Autodesk Fusion 360 part; units mm, degrees
(part 2 of 2)
  arc A403 (168.143, 73.5075) -> (169.394, 73.446) centre (168.77, 73.5075) ccw
  line L397 (168.143, 73.5075) -> (168.146, 74.619)
  circle A404 centre (161.56, 73.5325) radius 0.325
  circle A405 centre (167.34, 73.5325) radius 0.325
  arc A406 (174.75, 72.525) -> (175, 72.775) centre (174.75, 72.775) ccw
  line L398 (174.75, 72.525) -> (173.85, 72.525)
  arc A407 (173.6, 72.775) -> (173.85, 72.525) centre (173.85, 72.775) ccw
  line L399 (173.6, 72.775) -> (173.6, 73.3)
  arc A408 (173.85, 73.55) -> (173.6, 73.3) centre (173.85, 73.3) ccw
  line L400 (173.85, 73.55) -> (174.75, 73.55)
  arc A409 (175, 73.3) -> (174.75, 73.55) centre (174.75, 73.3) ccw
  line L401 (175, 73.3) -> (175, 72.775)
  arc A410 (157.05, 72.475) -> (157.3, 72.725) centre (157.05, 72.725) ccw
  line L402 (157.05, 72.475) -> (156.15, 72.475)
  arc A411 (155.9, 72.725) -> (156.15, 72.475) centre (156.15, 72.725) ccw
  line L403 (155.9, 72.725) -> (155.9, 73.25)
  arc A412 (156.15, 73.5) -> (155.9, 73.25) centre (156.15, 73.25) ccw
  line L404 (156.15, 73.5) -> (157.05, 73.5)
  arc A413 (157.3, 73.25) -> (157.05, 73.5) centre (157.05, 73.25) ccw
  line L405 (157.3, 73.25) -> (157.3, 72.725)
  arc A414 (174.775, 70) -> (175.025, 70.25) centre (174.775, 70.25) ccw
  line L406 (174.775, 70) -> (173.825, 70)
  arc A415 (173.575, 70.25) -> (173.825, 70) centre (173.825, 70.25) ccw
  line L407 (173.575, 70.25) -> (173.575, 70.75)
  arc A416 (173.825, 71) -> (173.575, 70.75) centre (173.825, 70.75) ccw
  line L408 (173.825, 71) -> (174.775, 71)
  arc A417 (175.025, 70.75) -> (174.775, 71) centre (174.775, 70.75) ccw
  line L409 (175.025, 70.75) -> (175.025, 70.25)
  arc A418 (160.632, 70.2525) -> (159.628, 70.2525) centre (160.13, 70.2525) ccw
  line L410 (160.632, 70.2525) -> (160.632, 69.4525)
  arc A419 (159.628, 69.4525) -> (160.632, 69.4525) centre (160.13, 69.4525) ccw
  line L411 (159.628, 69.4525) -> (159.628, 70.2525)
  arc A420 (169.272, 70.2525) -> (168.268, 70.2525) centre (168.77, 70.2525) ccw
  line L412 (169.272, 70.2525) -> (169.272, 69.4525)
  arc A421 (168.268, 69.4525) -> (169.272, 69.4525) centre (168.77, 69.4525) ccw
  line L413 (168.268, 69.4525) -> (168.268, 70.2525)
  arc A422 (174.775, 68.1) -> (175.025, 68.35) centre (174.775, 68.35) ccw
  line L414 (174.775, 68.1) -> (173.825, 68.1)
  arc A423 (173.575, 68.35) -> (173.825, 68.1) centre (173.825, 68.35) ccw
  line L415 (173.575, 68.35) -> (173.575, 68.85)
  arc A424 (173.825, 69.1) -> (173.575, 68.85) centre (173.825, 68.85) ccw
  line L416 (173.825, 69.1) -> (174.775, 69.1)
  arc A425 (175.025, 68.85) -> (174.775, 69.1) centre (174.775, 68.85) ccw
  line L417 (175.025, 68.85) -> (175.025, 68.35)
  line L418 (220, 60) -> (110, 60)
  line L419 (110, 60) -> (110, 170)
  line L420 (110, 170) -> (220, 170)
  line L421 (220, 170) -> (220, 60)
  line L422 (220, 60) -> (110, 170) construction
  line L423 (110, 60) -> (220, 170) construction
  point P0 (165, 115)
  constraint horizontal L418
  constraint perpendicular L418 L419
  constraint parallel L418 L420
  constraint parallel L419 L421
  constraint coincident L422 P0
  constraint coincident L423 P0
extrude "Extrude1" add sketch "Sketch1" along normal blind 10 contours L418 L419 L420 L421
sketch "Sketch2" plane through (0, 0, -0.05) normal (0, 0, 1) x (-1, 0, 0)
  line L0 (-115.9, 71.8) -> (-115.9024, 71.5818)
  arc A0 (-120.6818, 66.8024) -> (-115.9024, 71.5818) centre (-120.9, 71.8) ccw
  line L1 (-120.6818, 66.8024) -> (-120.9, 66.8)
  line L2 (-120.9, 66.8) -> (-209.95, 66.8)
  line L3 (-209.95, 66.8) -> (-210.1682, 66.8024)
  arc A1 (-214.9476, 71.5818) -> (-210.1682, 66.8024) centre (-209.95, 71.8) ccw
  line L4 (-214.9476, 71.5818) -> (-214.95, 71.8)
  line L5 (-214.95, 71.8) -> (-214.95, 155.9)
  line L6 (-214.95, 155.9) -> (-214.9476, 156.1182)
  arc A2 (-210.1682, 160.8976) -> (-214.9476, 156.1182) centre (-209.95, 155.9) ccw
  line L7 (-210.1682, 160.8976) -> (-209.95, 160.9)
  line L8 (-209.95, 160.9) -> (-120.9, 160.9)
  line L9 (-120.9, 160.9) -> (-120.6818, 160.8976)
  arc A3 (-115.9024, 156.1182) -> (-120.6818, 160.8976) centre (-120.9, 155.9) ccw
  line L10 (-115.9024, 156.1182) -> (-115.9, 155.9)
  line L11 (-115.9, 155.9) -> (-115.9, 71.8)
  line L12 (-110, 170) -> (-220, 170)
  line L13 (-220, 170) -> (-220, 60)
  line L14 (-220, 60) -> (-110, 60)
  line L15 (-110, 60) -> (-110, 170)
  circle A4 centre (-122.6756, 73.6401) radius 7.5719
  circle A5 centre (-208.2, 73.5) radius 7.6609
  circle A6 centre (-211.7862, 157.3826) radius 8.1229
  circle A7 centre (-122.6, 154.1) radius 8.9766
extrude "Extrude2" add sketch "Sketch2" against normal blind 10 contours L0 A0 L1 L2 L11 A4 | L8 L9 A3 L10 L11 A7 | L2 L3 A1 L4 L5 A5 | L5 L6 A2 L7 L8 A6 picked at (-121.8657, 72.2322) picked at (-121.9336, 154.8688) picked at (-209.4122, 72.673) picked at (-210.1646, 156.3085)
sketch "Sketch3" plane through (0, 0, -10.05) normal (0, 0, -1) x (1, 0, 0)
  line L0 (115.9, 77.02) -> (115.9, 148.126)
  arc A0 (115.9, 148.126) -> (128.4599, 160.9) centre (122.6, 154.1) ccw
  line L1 (128.4599, 160.9) -> (204.4644, 160.9)
  arc A1 (204.4644, 160.9) -> (214.95, 149.9011) centre (211.7862, 157.3826) ccw
  line L2 (214.95, 149.9011) -> (214.95, 77.1232)
  arc A2 (214.95, 77.1232) -> (204.4852, 66.8) centre (208.2, 73.5) ccw
  line L3 (204.4852, 66.8) -> (125.9231, 66.8)
  arc A3 (125.9231, 66.8) -> (115.9, 77.02) centre (122.6756, 73.6401) ccw
  line L4 (220, 170) -> (110, 170)
  line L5 (110, 170) -> (110, 60)
  line L6 (110, 60) -> (220, 60)
  line L7 (220, 60) -> (220, 170)
sketch "Sketch4" plane through (0, 0, 1.56) normal (0, 0, 1) x (-1, 0, 0)
  arc A0 (-120.6818, 66.8024) -> (-115.9024, 71.5818) centre (-120.9, 71.8) ccw
  line L0 (-115.9024, 71.5818) -> (-115.9, 71.8)
  line L1 (-115.9, 71.8) -> (-115.9, 155.9)
  line L2 (-115.9, 155.9) -> (-115.9024, 156.1182)
  arc A1 (-115.9024, 156.1182) -> (-120.6818, 160.8976) centre (-120.9, 155.9) ccw
  line L3 (-120.6818, 160.8976) -> (-120.9, 160.9)
  line L4 (-120.9, 160.9) -> (-209.95, 160.9)
  line L5 (-209.95, 160.9) -> (-210.1682, 160.8976)
  arc A2 (-210.1682, 160.8976) -> (-214.9476, 156.1182) centre (-209.95, 155.9) ccw
  line L6 (-214.9476, 156.1182) -> (-214.95, 155.9)
  line L7 (-214.95, 155.9) -> (-214.95, 71.8)
  line L8 (-214.95, 71.8) -> (-214.9476, 71.5818)
  arc A3 (-214.9476, 71.5818) -> (-210.1682, 66.8024) centre (-209.95, 71.8) ccw
  line L9 (-210.1682, 66.8024) -> (-209.95, 66.8)
  line L10 (-209.95, 66.8) -> (-120.9, 66.8)
  line L11 (-120.9, 66.8) -> (-120.6818, 66.8024)
  circle A4 centre (-122.55, 154.05) radius 2.2
  circle A5 centre (-208.4, 153.95) radius 2.2
  circle A6 centre (-165.24, 143.58) radius 2
  circle A7 centre (-160.16, 143.58) radius 0.85
  circle A8 centre (-170.32, 143.58) radius 0.85
  circle A9 centre (-161.43, 141.04) radius 1.1
  circle A10 centre (-167.78, 138.5) radius 1.1
  arc A11 (-139.5592, 132.4456) -> (-139.2145, 132.4456) centre (-139.3868, 132.6179) ccw
  line L12 (-139.5592, 132.4456) -> (-140.2044, 133.0908)
  arc A12 (-140.2044, 133.4355) -> (-140.2044, 133.0908) centre (-140.0321, 133.2632) ccw
  line L13 (-140.2044, 133.4355) -> (-139.8597, 133.7802)
  arc A13 (-139.515, 133.7802) -> (-139.8597, 133.7802) centre (-139.6873, 133.6079) ccw
  line L14 (-139.515, 133.7802) -> (-138.8698, 133.135)
  arc A14 (-138.8698, 132.7903) -> (-138.8698, 133.135) centre (-139.0421, 132.9627) ccw
  line L15 (-138.8698, 132.7903) -> (-139.2145, 132.4456)
  arc A15 (-134.6092, 132.3956) -> (-134.2645, 132.3956) centre (-134.4368, 132.5679) ccw
  line L16 (-134.6092, 132.3956) -> (-135.2544, 133.0408)
  arc A16 (-135.2544, 133.3855) -> (-135.2544, 133.0408) centre (-135.0821, 133.2132) ccw
  line L17 (-135.2544, 133.3855) -> (-134.9097, 133.7302)
  arc A17 (-134.565, 133.7302) -> (-134.9097, 133.7302) centre (-134.7373, 133.5579) ccw
  line L18 (-134.565, 133.7302) -> (-133.9198, 133.085)
  arc A18 (-133.9198, 132.7403) -> (-133.9198, 133.085) centre (-134.0921, 132.9127) ccw
  line L19 (-133.9198, 132.7403) -> (-134.2645, 132.3956)
  arc A19 (-129.8592, 132.2456) -> (-129.5145, 132.2456) centre (-129.6868, 132.4179) ccw
  line L20 (-129.8592, 132.2456) -> (-130.5044, 132.8908)
  arc A20 (-130.5044, 133.2355) -> (-130.5044, 132.8908) centre (-130.3321, 133.0632) ccw
  line L21 (-130.5044, 133.2355) -> (-130.1597, 133.5802)
  arc A21 (-129.815, 133.5802) -> (-130.1597, 133.5802) centre (-129.9873, 133.4079) ccw
  line L22 (-129.815, 133.5802) -> (-129.1698, 132.935)
  arc A22 (-129.1698, 132.5903) -> (-129.1698, 132.935) centre (-129.3421, 132.7627) ccw
  line L23 (-129.1698, 132.5903) -> (-129.5145, 132.2456)
  arc A23 (-140.885, 131.1198) -> (-140.5403, 131.1198) centre (-140.7127, 131.2921) ccw
  line L24 (-140.885, 131.1198) -> (-141.5302, 131.765)
  arc A24 (-141.5302, 132.1097) -> (-141.5302, 131.765) centre (-141.3579, 131.9373) ccw
  line L25 (-141.5302, 132.1097) -> (-141.1855, 132.4544)
  arc A25 (-140.8408, 132.4544) -> (-141.1855, 132.4544) centre (-141.0132, 132.2821) ccw
  line L26 (-140.8408, 132.4544) -> (-140.1956, 131.8092)
  arc A26 (-140.1956, 131.4645) -> (-140.1956, 131.8092) centre (-140.3679, 131.6368) ccw
  line L27 (-140.1956, 131.4645) -> (-140.5403, 131.1198)
  arc A27 (-135.935, 131.0698) -> (-135.5903, 131.0698) centre (-135.7627, 131.2421) ccw
  line L28 (-135.935, 131.0698) -> (-136.5802, 131.715)
  arc A28 (-136.5802, 132.0597) -> (-136.5802, 131.715) centre (-136.4079, 131.8873) ccw
  line L29 (-136.5802, 132.0597) -> (-136.2355, 132.4044)
  arc A29 (-135.8908, 132.4044) -> (-136.2355, 132.4044) centre (-136.0632, 132.2321) ccw
  line L30 (-135.8908, 132.4044) -> (-135.2456, 131.7592)
  arc A30 (-135.2456, 131.4145) -> (-135.2456, 131.7592) centre (-135.4179, 131.5868) ccw
  line L31 (-135.2456, 131.4145) -> (-135.5903, 131.0698)
  arc A31 (-131.185, 130.9198) -> (-130.8403, 130.9198) centre (-131.0127, 131.0921) ccw
  line L32 (-131.185, 130.9198) -> (-131.8302, 131.565)
  arc A32 (-131.8302, 131.9097) -> (-131.8302, 131.565) centre (-131.6579, 131.7373) ccw
  line L33 (-131.8302, 131.9097) -> (-131.4855, 132.2544)
  arc A33 (-131.1408, 132.2544) -> (-131.4855, 132.2544) centre (-131.3132, 132.0821) ccw
  line L34 (-131.1408, 132.2544) -> (-130.4956, 131.6092)
  arc A34 (-130.4956, 131.2645) -> (-130.4956, 131.6092) centre (-130.6679, 131.4368) ccw
  line L35 (-130.4956, 131.2645) -> (-130.8403, 130.9198)
  circle A35 centre (-155.356, 124.5071) radius 2
  circle A36 centre (-174.4162, 124.5068) radius 2
  circle A37 centre (-150.276, 124.5071) radius 0.85
  circle A38 centre (-160.436, 124.5071) radius 0.85
  circle A39 centre (-169.3362, 124.5068) radius 0.85
  circle A40 centre (-179.4962, 124.5068) radius 0.85
  circle A41 centre (-151.546, 121.9671) radius 1.1
  circle A42 centre (-170.6062, 121.9668) radius 1.1
  circle A43 centre (-157.896, 119.4271) radius 1.1
  circle A44 centre (-176.9562, 119.4268) radius 1.1
  circle A45 centre (-193.5, 115.37) radius 2
  circle A46 centre (-136.34, 114.88) radius 2
  circle A47 centre (-188.42, 115.37) radius 0.85
  circle A48 centre (-198.58, 115.37) radius 0.85
  circle A49 centre (-131.26, 114.88) radius 0.85
  circle A50 centre (-141.42, 114.88) radius 0.85
  circle A51 centre (-189.69, 112.83) radius 1.1
  circle A52 centre (-132.53, 112.34) radius 1.1
  circle A53 centre (-196.04, 110.29) radius 1.1
  circle A54 centre (-138.88, 109.8) radius 1.1
  circle A55 centre (-155.36, 105.48) radius 2
  circle A56 centre (-174.41, 105.48) radius 2
  circle A57 centre (-150.28, 105.48) radius 0.85
  circle A58 centre (-160.44, 105.48) radius 0.85
  circle A59 centre (-169.33, 105.48) radius 0.85
  circle A60 centre (-179.49, 105.48) radius 0.85
  circle A61 centre (-151.55, 102.94) radius 1.1
  circle A62 centre (-170.6, 102.94) radius 1.1
  circle A63 centre (-157.9, 100.4) radius 1.1
  circle A64 centre (-176.95, 100.4) radius 1.1
  line L36 (-196.9, 93.25) -> (-196.9, 95.25)
  line L37 (-196.9, 95.25) -> (-193.7, 95.25)
  line L38 (-193.7, 95.25) -> (-193.7, 93.25)
  line L39 (-193.7, 93.25) -> (-196.9, 93.25)
  circle A65 centre (-187.8, 91.15) radius 1
  circle A66 centre (-202.3, 91.15) radius 1
  circle A67 centre (-187.8, 88.65) radius 1
  circle A68 centre (-164.94, 86.38) radius 2
  circle A69 centre (-159.86, 86.38) radius 0.85
  circle A70 centre (-170.02, 86.38) radius 0.85
  line L40 (-188.8, 85.15) -> (-188.8, 87.15)
  line L41 (-188.8, 87.15) -> (-186.8, 87.15)
  line L42 (-186.8, 87.15) -> (-186.8, 85.15)
  line L43 (-186.8, 85.15) -> (-188.8, 85.15)
  circle A71 centre (-202.3, 86.15) radius 1
  circle A72 centre (-161.13, 83.84) radius 1.1
  line L44 (-196.9, 82.05) -> (-196.9, 84.05)
  line L45 (-196.9, 84.05) -> (-193.7, 84.05)
  line L46 (-193.7, 84.05) -> (-193.7, 82.05)
  line L47 (-193.7, 82.05) -> (-196.9, 82.05)
  circle A73 centre (-167.48, 81.3) radius 1.1
  circle A74 centre (-122.55, 73.65) radius 2.2
  circle A75 centre (-208.15, 73.55) radius 2.2
  arc A76 (-159.506, 74.619) -> (-160.757, 74.5575) centre (-160.13, 74.5575) ccw
  line L48 (-159.506, 74.619) -> (-159.503, 73.5075)
  arc A77 (-160.754, 73.446) -> (-159.503, 73.5075) centre (-160.13, 73.5075) ccw
  line L49 (-160.754, 73.446) -> (-160.757, 74.5575)
  arc A78 (-168.146, 74.619) -> (-169.397, 74.5575) centre (-168.77, 74.5575) ccw
  line L50 (-168.146, 74.619) -> (-168.143, 73.5075)
  arc A79 (-169.394, 73.446) -> (-168.143, 73.5075) centre (-168.77, 73.5075) ccw
  line L51 (-169.394, 73.446) -> (-169.397, 74.5575)
  circle A80 centre (-161.56, 73.5325) radius 0.325
  circle A81 centre (-167.34, 73.5325) radius 0.325
  arc A82 (-159.628, 70.2525) -> (-160.632, 70.2525) centre (-160.13, 70.2525) ccw
  line L52 (-159.628, 70.2525) -> (-159.628, 69.4525)
  arc A83 (-160.632, 69.4525) -> (-159.628, 69.4525) centre (-160.13, 69.4525) ccw
  line L53 (-160.632, 69.4525) -> (-160.632, 70.2525)
  arc A84 (-168.268, 70.2525) -> (-169.272, 70.2525) centre (-168.77, 70.2525) ccw
  line L54 (-168.268, 70.2525) -> (-168.268, 69.4525)
  arc A85 (-169.272, 69.4525) -> (-168.268, 69.4525) centre (-168.77, 69.4525) ccw
  line L55 (-169.272, 69.4525) -> (-169.272, 70.2525)
  circle A86 centre (-122.55, 73.65) radius 0.85
  circle A87 centre (-208.15, 73.55) radius 0.85
  circle A88 centre (-208.4, 153.95) radius 0.85
  circle A89 centre (-122.55, 154.05) radius 0.85
  dimension "d5" = 1.7
  dimension "d6" = 1.7
  dimension "d7" = 1.7
  dimension "d8" = 1.7
  constraint concentric A74 A86
  constraint concentric A75 A87
  constraint concentric A5 A88
  constraint concentric A4 A89
  measures "d5" diameter of A86
  measures "d6" diameter of A87
  measures "d7" diameter of A88
  measures "d8" diameter of A89
extrude "Extrude3" cut sketch "Sketch4" against normal blind 20 contours A86 | A87 | A88 | A89
sketch "Sketch5" plane through (0, 0, -0.05) normal (0, 0, 1) x (-1, 0, 0)
  line L0 (-110, 170) -> (-220, 170)
  line L1 (-220, 170) -> (-220, 60)
  line L2 (-220, 60) -> (-110, 60)
  line L3 (-110, 60) -> (-110, 170)
  arc A0 (-115.9, 77.02) -> (-125.9231, 66.8) centre (-122.6756, 73.6401) ccw
  line L4 (-125.9231, 66.8) -> (-204.4852, 66.8)
  arc A1 (-204.4852, 66.8) -> (-214.95, 77.1232) centre (-208.2, 73.5) ccw
  line L5 (-214.95, 77.1232) -> (-214.95, 149.9011)
  arc A2 (-214.95, 149.9011) -> (-204.4644, 160.9) centre (-211.7862, 157.3826) ccw
  line L6 (-204.4644, 160.9) -> (-128.4599, 160.9)
  arc A3 (-128.4599, 160.9) -> (-115.9, 148.126) centre (-122.6, 154.1) ccw
  line L7 (-115.9, 148.126) -> (-115.9, 77.02)
  circle A4 centre (-122.55, 154.05) radius 0.85
  circle A5 centre (-122.55, 73.65) radius 0.85
  circle A6 centre (-208.4, 153.95) radius 0.85
  circle A7 centre (-208.15, 73.55) radius 0.85
sketch "Sketch6" plane through (0, -60, 0) normal (0, 1, 0) x (-1, 0, 0)
  line L0 (-110, -0.05) -> (-220, -0.05)
  line L1 (-220, -0.05) -> (-220, -10.05)
  line L2 (-220, -10.05) -> (-110, -10.05)
  line L3 (-110, -10.05) -> (-110, -0.05)
  line L4 (-169.5053, -0.05) -> (-159.5, -0.05)
  line L5 (-159.5, -0.05) -> (-159.5, -16.5)
  line L6 (-159.5, -16.5) -> (-169.5053, -16.5)
  line L7 (-169.5053, -16.5) -> (-169.5053, -0.05)
  constraint horizontal L4
  constraint vertical L5
  constraint horizontal L6
  constraint vertical L7
  constraint coincident L0 L4.start
extrude "Extrude4" cut sketch "Sketch6" against normal blind 14 contours L0 L2 L4 L5 L7
extrude "Extrude5" add 1 faces at (169.5053, -64.5333, -3.3833) along direction (-1, 0, 0) blind 10
extrude "Extrude6" cut 2 faces at (199.8351, -60, -6.7167) (126.5, -60, -6.7167) along direction (0, -1, 0) blind 5
sketch "Sketch7" plane through (0, -65, 0) normal (0, 1, 0) x (-1, 0, 0)
  line L0 (-159.5053, -0.05) -> (-220, -0.05)
  line L1 (-220, -0.05) -> (-220, -10.05)
  line L2 (-220, -10.05) -> (-159.5053, -10.05)
  line L3 (-159.5053, -10.05) -> (-159.5053, -0.05)
  line L4 (-170.2701, -0.05) -> (-158.7543, -0.05)
  line L5 (-158.7543, -0.05) -> (-158.7543, -4.38)
  line L6 (-158.7543, -4.38) -> (-170.2701, -4.38)
  line L7 (-170.2701, -4.38) -> (-170.2701, -0.05)
  constraint horizontal L4
  constraint vertical L5
  constraint horizontal L6
  constraint vertical L7
  constraint coincident L0 L4.start
extrude "Extrude7" cut sketch "Sketch7" against normal blind 2 contours L0 L3 L4 L6 L7 | L3 L4 L5 L6
sketch "Sketch8" plane through (0, -170, 0) normal (0, -1, 0) x (1, 0, 0)
  line L0 (220, -0.05) -> (110, -0.05)
  line L1 (110, -0.05) -> (110, -10.05)
  line L2 (110, -10.05) -> (220, -10.05)
  line L3 (220, -10.05) -> (220, -0.05)
fillet "Fillet1" radius 7.5 1 edges at (220, -170, -5.05)
fillet "Fillet2" radius 7.5 3 edges at (110, -170, -5.05) (220, -65, -5.05) (110, -65, -5.05)
fillet "Fillet3" radius 1 2 edges at (158.7543, -65.9, -0.05) (170.2701, -65.9, -0.05)
